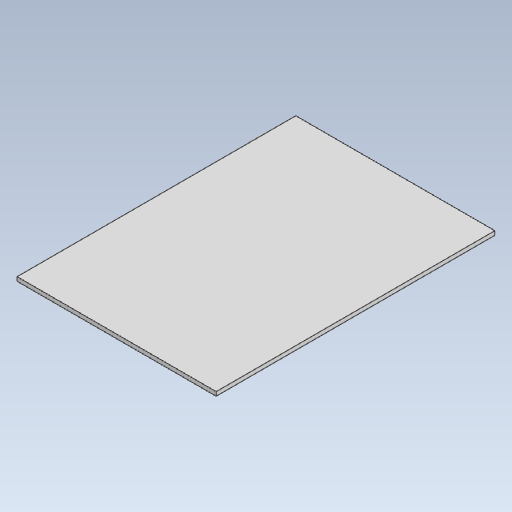
# Autodesk Inventor part: lower casing
Saved by Autodesk Inventor 2020 (Build 240168000, 168)
## iProperties
Created: 2019-06-23
Part Number: lower casing
Material: Generic
Document SubType Name: Modeling
Designer: jjsch
Density: 1 g/cm^3
Appearance: Default
Mass: 48.384 g
Surface Area: 417.024 cm^2
Volume: 48.384 cm^3
Author: jjsch
Autodesk Inventor part; units mm, degrees
ref_plane "YZ Plane" through (0, 0, 0) normal (1, 0, 0) x (0, 1, 0)
ref_plane "XZ Plane" through (0, 0, 0) normal (0, 1, 0) x (-1, 0, 0)
ref_plane "XY Plane" through (0, 0, 0) normal (0, 0, 1) x (1, 0, 0)
sketch "Sketch1" plane through (0, 0, 0) normal (0, 1, 0) x (-1, 0, 0)
  line L0 (-60, -84) -> (60, -84)
  line L1 (60, -84) -> (60, 84)
  line L2 (60, 84) -> (-60, 84)
  line L3 (-60, 84) -> (-60, -84)
  line L4 (-60, -84) -> (60, 84) construction
  line L5 (60, -84) -> (-60, 84) construction
  point P0 (0, 0)
  dimension "d0" = 168
  dimension "d1" = 120
  constraints: 12 end point, 2 midpoint, 2 parallel, 1 horizontal, 1 perpendicular
  measures "d0" distance of L1.end L0.end
  measures "d1" distance of L1.end L2.end
extrude "Extrusion1" add sketch "Sketch1" along normal blind 2.4
body "Solid1"
